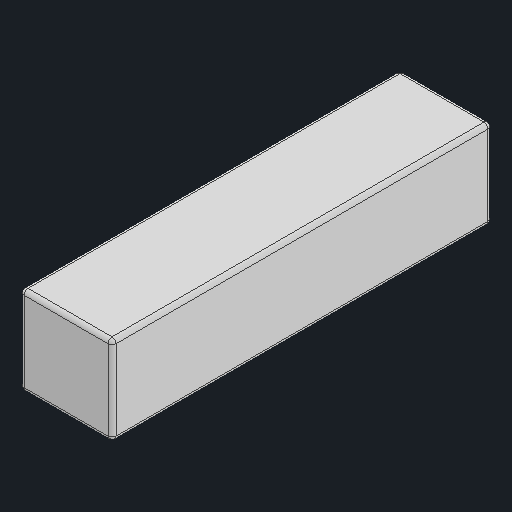
# Autodesk Inventor part: Battery_Small
Saved by Autodesk Inventor 2026.2 (Build 302298000, 298)
## iProperties
Created: 2026-02-03
Part Number: Battery_Small
Material: Generic
Document SubType Name: Modeling
Designer: vckot
Density: 1 g/cm^3
Appearance: Default
Author: vckot
Autodesk Inventor part; units mm, degrees
ref_plane "YZ Plane" through (0, 0, 0) normal (1, 0, 0) x (0, 1, 0)
ref_plane "XZ Plane" through (0, 0, 0) normal (0, 1, 0) x (-1, 0, 0)
ref_plane "XY Plane" through (0, 0, 0) normal (0, 0, 1) x (1, 0, 0)
sketch "Sketch1" plane through (0, 0, 0) normal (0, 1, 0) x (-1, 0, 0)
  line L0 (-11.5, 47.5) -> (11.5, 47.5)
  line L1 (11.5, 47.5) -> (11.5, -47.5)
  line L2 (11.5, -47.5) -> (-11.5, -47.5)
  line L3 (-11.5, -47.5) -> (-11.5, 47.5)
  line L4 (-11.5, 47.5) -> (11.5, -47.5) construction
  line L5 (11.5, 47.5) -> (-11.5, -47.5) construction
  point P0 (0, 0)
  dimension "d0" = 95
  dimension "d1" = 23
  constraints: 12 end point, 2 midpoint, 2 parallel, 1 horizontal, 1 perpendicular
  measures "d0" distance of L0.end L1.end
  measures "d1" distance of L1.end L2.end
extrude "Extrusion1" add sketch "Sketch1" along normal mid plane 22
fillet "Fillet1" radius 1 12 edges at (0, 11, 47.5) (11.5, 11, 0) (11.5, 0, 47.5) (-11.5, 0, 47.5) (11.5, -11, 0) (0, -11, 47.5) (-11.5, 11, 0) (-11.5, -11, 0) (0, 11, -47.5) (-11.5, 0, -47.5) (11.5, 0, -47.5) (0, -11, -47.5)
body "Solid1"
